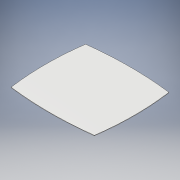
# Autodesk Inventor part: kawa
Saved by Autodesk Inventor 2019 (Build 230136000, 136)
## iProperties
Created: 2019-11-16
Part Number: kawa
Material: Кожа, темно-коричневая
Document SubType Name: Modeling
Designer: stepa
Density: 0.9 g/cm^3
Appearance: Белый
Author: stepa
Autodesk Inventor part; units mm, degrees
ref_plane "YZ Plane" through (0, 0, 0) normal (1, 0, 0) x (0, 1, 0)
ref_plane "XZ Plane" through (0, 0, 0) normal (0, 1, 0) x (-1, 0, 0)
ref_plane "XY Plane" through (0, 0, 0) normal (0, 0, 1) x (1, 0, 0)
sketch "Эскиз1" plane through (0, 0, 0) normal (0, 1, 0) x (-1, 0, 0)
  line L0 (0, -200) -> (-220, -200)
  line L1 (-220, -200) -> (-220, 0)
  line L2 (-220, 0) -> (0, 0)
  line L3 (0, 0) -> (0, -200)
  line L4 (-30, -170) -> (-190, -170)
  line L5 (-190, -170) -> (-190, -30)
  line L6 (-190, -30) -> (-30, -30)
  line L7 (-30, -30) -> (-30, -170)
  line L8 (0, -200) -> (-30, -170)
  line L9 (-220, -200) -> (-190, -170)
  line L10 (0, 0) -> (-30, -30)
  line L11 (-220, 0) -> (-190, -30)
  line L12 (-30, -170) -> (-15.8579, -184.1421)
  line L13 (-190, -170) -> (-204.1421, -184.1421)
  line L14 (-190, -30) -> (-204.1421, -15.8579)
  line L15 (-30, -30) -> (-15.8579, -15.8579)
  arc A0 (-204.1421, -184.1421) -> (-15.8579, -184.1421) centre (-110, 569.4113) ccw
  arc A1 (-15.8579, -184.1421) -> (-15.8579, -15.8579) centre (-617.2361, -100) ccw
  arc A2 (-204.1421, -15.8579) -> (-204.1421, -184.1421) centre (397.2361, -100) ccw
  arc A3 (-15.8579, -15.8579) -> (-204.1421, -15.8579) centre (-110, -769.4113) ccw
  point P0 (-110, -190)
  point P1 (-10, -100)
  point P2 (-210, -100)
  point P3 (-110, -10)
  dimension "d0" = 220
  dimension "d1" = 200
  dimension "d2" = 30
  dimension "d3" = 30
  dimension "d4" = 30
  dimension "d5" = 30
  dimension "d6" = 20
  dimension "d7" = 20
  dimension "d8" = 20
  dimension "d9" = 20
  dimension "d10" = 20
  dimension "d11" = 20
  dimension "d12" = 20
  dimension "d13" = 20
  constraints: 32 end point, 12 point on circle, 4 centre point, 4 parallel, 4 point on line, 2 horizontal, 2 perpendicular, 1 coincident
  measures "d0" distance of L1.end L2.end
  measures "d1" distance of L0.end L1.end
  measures "d2" distance between parallel lines of L0 L4
  measures "d3" distance between parallel lines of L1 L5
  measures "d4" distance between parallel lines of L2 L6
  measures "d5" distance between parallel lines of L3 L7
  measures "d6" distance of L4.start L12.end
  measures "d7" distance of L4.end L13.end
  measures "d8" distance of L5.end L14.end
  measures "d9" distance of L6.end L15.end
  measures "d10" distance from line of L4 point (-110, -190)
  measures "d11" distance from line of L7 point (-10, -100)
  measures "d12" distance from line of L5 point (-210, -100)
  measures "d13" distance from line of L6 point (-110, -10)
extrude "Выдавливание1" add sketch "Эскиз1" along normal blind 1 contours A0 L9 L4 L8 | L8 L7 L10 A1 | A2 L11 L5 L9 | L10 L6 L11 A3 | L4 L5 L6 L7
